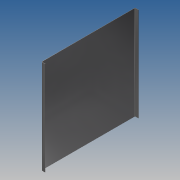
# Autodesk Inventor part: DD_KVD_002_02
Saved by Autodesk Inventor 2017.3 (Build 213256000, 256)
## iProperties
Created: 2023-12-04
Part Number: DD_KVD_002_02
Material: Nerezová ocel
Document SubType Name: Sheet Metal
Designer: Darena
Density: 8 g/cm^3
Flat Pattern Width: 80 cm
Flat Pattern Length: 85.1305 cm
Flat Pattern Area: 6810.44 cm^2
Sheet Metal Rule: Výchozí_mm
Sheet Metal Width: 800,000 mm
Sheet Metal Length: 851,305 mm
Sheet Metal Area: 681044,246 mm^2
Appearance: Pololeštěná
Author: Darena
Title: DÍL SVAŘENCE - 08
Autodesk Inventor part; units mm, degrees
ref_plane "YZ Plane" through (0, 0, 0) normal (1, 0, 0) x (0, 1, 0)
ref_plane "XZ Plane" through (0, 0, 0) normal (0, 1, 0) x (-1, 0, 0)
ref_plane "XY Plane" through (0, 0, 0) normal (0, 0, 1) x (1, 0, 0)
sketch "Náčrt2" plane through (0, 0, 0) normal (1, 0, 0) x (0, 1, 0)
  line L0 (800, 400) -> (0, 400)
  line L1 (0, 400) -> (0, -400)
  line L2 (0, -400) -> (800, -400)
  line L3 (800, -400) -> (800, 400)
  point P0 (0, 0)
  point P1 (0, 0)
  dimension "d0" = 800
  dimension "d1" = 800
  constraints: 8 end point, 2 coincident, 2 parallel, 1 horizontal, 1 midpoint, 1 perpendicular
  measures "d0" distance of L0.end L1.end
  measures "d1" distance of L0.start L0.end
extrude "Vysunutí1" add sketch "Náčrt2" against normal blind 2.5
sketch "Náčrt3" plane through (-2.5, 797.5, 400) normal (0, 1, 0) x (-1, 0, 0)
  line L0 (0, -800) -> (0, 0)
  line L1 (0, 0) -> (-31.5, 0)
  line L2 (-31.5, 0) -> (-31.5, -800)
  line L3 (-31.5, -800) -> (0, -800)
  constraints: 6 end point, 1 horizontal, 1 perpendicular, 1 vertical
edge flange "Obruba1" height 31.5 angle 90 thickness 2.5 bend radius 6 thickness toward (0, 1, 0) relief tear relief width 2.5 relief depth 1.25 corner gap 2.5 corner form 0 edges at (0, 800, 0) (0, 0, 0) wall of the first edge with corners at (-2.5, 797.5, -400) (-2.5, 797.5, 400) (29, 797.5, 400) (29, 797.5, -400)
bend "Ohyb1"
corner "Roh1"
equation "\"d4\" = ŠířkaVýštipu"
equation "\"d5\" = HloubkaVýštipu"
equation "\"d6\" = MinimálníZbytek"
equation "\"d7\" = PoloměrOhybu"
equation "\"d11\" = VelikostRohovéhoVýštipu"
equation "\"d12\" = VelikostMezery"
equation "\"d13\" = VelikostJacobihoPoloměru"
equation "\"PoloměrOhybu\" = Tloušťka"
equation "\"ŠířkaVýštipu\" = Tloušťka"
equation "\"HloubkaVýštipu\" = 0.5 * Tloušťka"
equation "\"MinimálníZbytek\" = 2 * Tloušťka"
equation "\"PřechodovýPoloměr\" = PoloměrOhybu"
equation "\"VelikostJacobihoPoloměru\" = PoloměrOhybu"
equation "\"VelikostMezery\" = Tloušťka"
equation "\"VelikostRohovéhoVýštipu\" = 10"
equation "\"Tloušťka\" = 2.5"
